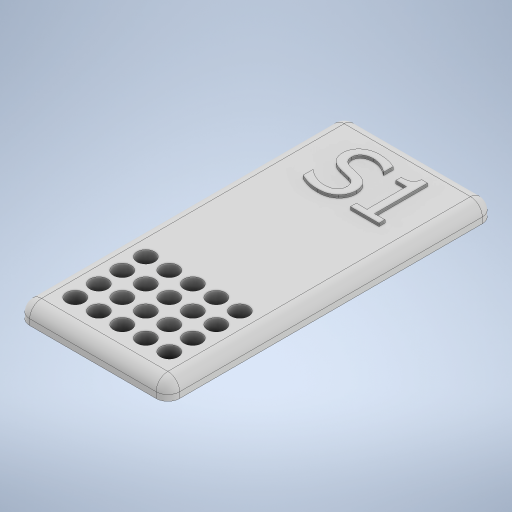
# Autodesk Inventor part: sensor1
Saved by Autodesk Inventor 2024 (Build 280153000, 153)
## iProperties
Created: 2024-03-11
Part Number: sensor1
Material: Generic
Document SubType Name: Modeling
Designer: quinten
Density: 1 g/cm^3
Appearance: Default
Author: quinten
Autodesk Inventor part; units mm, degrees
ref_plane "YZ Plane" through (0, 0, 0) normal (1, 0, 0) x (0, 1, 0)
ref_plane "XZ Plane" through (0, 0, 0) normal (0, 1, 0) x (-1, 0, 0)
ref_plane "XY Plane" through (0, 0, 0) normal (0, 0, 1) x (1, 0, 0)
sketch "Sketch1" plane through (0, 0, 0) normal (0, 1, 0) x (-1, 0, 0)
  line L0 (0, 0) -> (21.5, 0)
  line L1 (21.5, 0) -> (21.5, -51.5)
  line L2 (21.5, -51.5) -> (0, -51.5)
  line L3 (0, -51.5) -> (0, 0)
  line L4 (23.5, 2) -> (-2, 2)
  line L5 (-2, 2) -> (-2, -53.5)
  line L6 (-2, -53.5) -> (23.5, -53.5)
  line L7 (23.5, -53.5) -> (23.5, 2)
  line L8 (10.75, 0) -> (10.75, -51.5) construction
  circle A0 centre (10.75, -3) radius 1.5
  line L9 (0, -3) -> (21.5, -3) construction
  circle A1 centre (14.75, -3) radius 1.5
  circle A2 centre (18.75, -3) radius 1.5
  circle A3 centre (6.75, -3) radius 1.5
  circle A4 centre (2.75, -3) radius 1.5
  circle A5 centre (18.75, -7) radius 1.5
  circle A6 centre (14.75, -7) radius 1.5
  circle A7 centre (10.75, -7) radius 1.5
  circle A8 centre (6.75, -7) radius 1.5
  circle A9 centre (2.75, -7) radius 1.5
  circle A10 centre (18.75, -11) radius 1.5
  circle A11 centre (14.75, -11) radius 1.5
  circle A12 centre (10.75, -11) radius 1.5
  circle A13 centre (6.75, -11) radius 1.5
  circle A14 centre (2.75, -11) radius 1.5
  circle A15 centre (18.75, -15) radius 1.5
  circle A16 centre (14.75, -15) radius 1.5
  circle A17 centre (10.75, -15) radius 1.5
  circle A18 centre (6.75, -15) radius 1.5
  circle A19 centre (2.75, -15) radius 1.5
  point P0 (10.75, -3)
  point P1 (10.75, -7)
  point P2 (10.75, -11)
  point P3 (10.75, -15)
  dimension "d0" = 21.5
  dimension "d1" = 51.5
  dimension "d2" = 2
  dimension "d3" = 2
  dimension "d4" = 2
  dimension "d5" = 2
  dimension "d6" = 3
  dimension "d8" = 3
  dimension "d9" = 3
  dimension "d10" = 3
  dimension "d11" = 3
  dimension "d12" = 3
  dimension "d13" = 4
  dimension "d14" = 4
  dimension "d15" = 4
  dimension "d16" = 4
  dimension "d19" = 4
  constraints: 20 centre point, 20 end point, 7 point on line, 4 midpoint, 4 parallel, 3 perpendicular, 2 horizontal, 1 vertical, 33 other
  measures "d0" distance of L1.end L2.end
  measures "d1" distance of L0.end L1.end
  measures "d2" distance between parallel lines of L7 L1
  measures "d3" distance between parallel lines of L0 L4
  measures "d4" distance between parallel lines of L3 L5
  measures "d5" distance between parallel lines of L6 L2
  measures "d6" diameter of A0
  measures "d8" distance between parallel lines of L0 L9
  measures "d9" diameter of A1
  measures "d10" diameter of A2
  measures "d11" diameter of A3
  measures "d12" diameter of A4
  measures "d13" distance of point (10.75, -3) A3.centre
  measures "d14" distance of A3.centre A4.centre
  measures "d15" distance of A1.centre point (10.75, -3)
  measures "d16" distance of A2.centre A1.centre
  measures "d19" distance of A2.centre A5.centre
extrude "Extrusion1" add sketch "Sketch1" along normal blind 3 contours L0 L1 L2 L3 | L7 L6 L5 L4
fillet "Fillet1" radius 2 8 edges at (-23.5, 3, -25.75) (-10.75, 3, 2) (-23.5, 1.5, 2) (2, 1.5, 2) (2, 3, -25.75) (-10.75, 3, -53.5) (-23.5, 1.5, -53.5) (2, 1.5, -53.5)
sketch "Sketch2" plane through (0, 3, 0) normal (0, 1, 0) x (1, 0, 0)
  line L0 (-17.4247, 49.4836) -> (-8.1758, 49.4836) construction
  line L1 (-8.1758, 49.4836) -> (-8.1758, 43.1661) construction
  line L2 (-8.1758, 43.1661) -> (-17.4247, 43.1661) construction
  line L3 (-17.4247, 43.1661) -> (-17.4247, 49.4836) construction
  spline S0 degree 2 poles (-13.624, 39.127) (-14.7099, 39.127) (-16.2334, 39.5808) (-16.906, 39.905) knots 0 0 0 1 2 2 2
  line L4 (-16.906, 39.905) -> (-16.906, 41.5744)
  line L5 (-16.906, 41.5744) -> (-16.8088, 41.5744)
  spline S1 degree 2 poles (-16.8088, 41.5744) (-16.1524, 40.9585) (-14.4911, 40.2778) (-13.7213, 40.2778) knots 0 0 0 1 2 2 2
  spline S2 degree 2 poles (-13.7213, 40.2778) (-12.6192, 40.2778) (-11.4928, 41.1935) (-11.4928, 41.9471) knots 0 0 0 1 2 2 2
  spline S3 degree 2 poles (-11.4928, 41.9471) (-11.4928, 42.5468) (-12.0843, 43.2923) (-12.7245, 43.4787) knots 0 0 0 1 2 2 2
  spline S4 degree 2 poles (-12.7245, 43.4787) (-13.1864, 43.6084) (-13.9563, 43.7867) (-14.5317, 43.9325) knots 0 0 0 1 2 2 2
  spline S5 degree 2 poles (-14.5317, 43.9325) (-15.0503, 44.0703) (-15.8688, 44.4836) (-16.1848, 44.8158) knots 0 0 0 1 2 2 2
  spline S6 degree 2 poles (-16.1848, 44.8158) (-16.4928, 45.1481) (-16.8331, 46.0395) (-16.8331, 46.623) knots 0 0 0 1 2 2 2
  spline S7 degree 2 poles (-16.8331, 46.623) (-16.8331, 47.8385) (-14.9368, 49.4836) (-13.4701, 49.4836) knots 0 0 0 1 2 2 2
  spline S8 degree 2 poles (-13.4701, 49.4836) (-12.6273, 49.4836) (-11.1362, 49.1513) (-10.496, 48.8353) knots 0 0 0 1 2 2 2
  line L6 (-10.496, 48.8353) -> (-10.496, 47.247)
  line L7 (-10.496, 47.247) -> (-10.5932, 47.247)
  spline S9 degree 2 poles (-10.5932, 47.247) (-11.0714, 47.6846) (-12.5624, 48.3329) (-13.3809, 48.3329) knots 0 0 0 1 2 2 2
  spline S10 degree 2 poles (-13.3809, 48.3329) (-14.3047, 48.3329) (-15.4474, 47.4658) (-15.4474, 46.7607) knots 0 0 0 1 2 2 2
  spline S11 degree 2 poles (-15.4474, 46.7607) (-15.4474, 46.1287) (-14.7748, 45.375) (-14.1427, 45.2048) knots 0 0 0 1 2 2 2
  spline S12 degree 2 poles (-14.1427, 45.2048) (-13.7213, 45.0914) (-12.4976, 44.7996) (-12.0924, 44.6781) knots 0 0 0 1 2 2 2
  spline S13 degree 2 poles (-12.0924, 44.6781) (-11.0633, 44.362) (-10.107, 43.0898) (-10.107, 42.1578) knots 0 0 0 1 2 2 2
  spline S14 degree 2 poles (-10.107, 42.1578) (-10.107, 41.5663) (-10.5851, 40.4317) (-11.0146, 40.0346) knots 0 0 0 1 2 2 2
  spline S15 degree 2 poles (-11.0146, 40.0346) (-11.4928, 39.597) (-12.7083, 39.127) (-13.624, 39.127) knots 0 0 0 1 2 2 2
  line L8 (-3.3728, 39.3053) -> (-8.2513, 39.3053)
  line L9 (-8.2513, 39.3053) -> (-8.2513, 40.3264)
  line L10 (-8.2513, 40.3264) -> (-6.436, 40.3264)
  line L11 (-6.436, 40.3264) -> (-6.436, 47.0282)
  line L12 (-6.436, 47.0282) -> (-8.2513, 47.0282)
  line L13 (-8.2513, 47.0282) -> (-8.2513, 47.9439)
  spline S16 degree 2 poles (-8.2513, 47.9439) (-7.2221, 47.9439) (-6.2496, 48.5274) (-6.1848, 49.3377) knots 0 0 0 1 2 2 2
  line L14 (-6.1848, 49.3377) -> (-5.1475, 49.3377)
  line L15 (-5.1475, 49.3377) -> (-5.1475, 40.3264)
  line L16 (-5.1475, 40.3264) -> (-3.3728, 40.3264)
  line L17 (-3.3728, 40.3264) -> (-3.3728, 39.3053)
  point P0 (0, 0)
  constraints: 2 other
extrude "Extrusion2" add sketch "Sketch2" along normal blind 0.5
equation "\"d8\" = d6"
equation "\"d9\" = d11"
equation "\"d10\" = d11"
equation "\"d11\" = d6"
equation "\"d12\" = d11"
equation "\"d14\" = d13"
equation "\"d15\" = d13"
equation "\"d16\" = d15"
body "Solid1"
